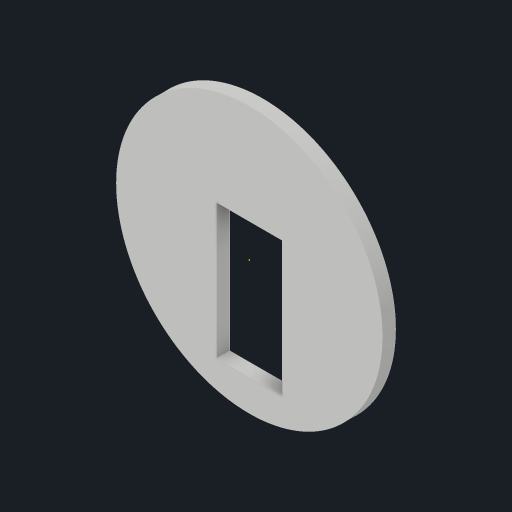
# Autodesk Inventor part: base22
Saved by Autodesk Inventor 2023.4 (Build 274418000, 418)
## iProperties
Created: 2016-02-08
Part Number: base22
Material: Generic
Document SubType Name: Modeling
Designer: Nanjar
Density: 1 g/cm^3
Appearance: Default
Author: Nanjar
Autodesk Inventor part; units mm, degrees
ref_plane "YZ Plane" through (0, 0, 0) normal (1, 0, 0) x (0, 1, 0)
ref_plane "XZ Plane" through (0, 0, 0) normal (0, 1, 0) x (-1, 0, 0)
ref_plane "XY Plane" through (0, 0, 0) normal (0, 0, 1) x (1, 0, 0)
sketch "Sketch1" plane through (0, 0, 0) normal (0, 0, 1) x (1, 0, 0)
  circle A0 centre (0, 0) radius 40
  circle A1 centre (0, 0) radius 5.375
  dimension "d0" = 80
  dimension "d1" = 10.75
  constraints: 2 centre point, 2 coincident
  measures "d0" diameter of A0
  measures "d1" diameter of A1
extrude "Extrusion1" add sketch "Sketch1" along normal blind 4
sketch "Sketch5" plane through (0, 0, 4) normal (0, 0, 1) x (1, 0, 0)
  point P0 (0, 0)
sketch "Sketch7" plane through (0, 0, 4) normal (0, 0, 1) x (1, 0, 0)
  line L0 (-9.9, 10) -> (9.9, 10)
  line L1 (9.9, 10) -> (9.9, -30.6)
  line L2 (9.9, -30.6) -> (-9.9, -30.6)
  line L3 (-9.9, -30.6) -> (-9.9, 10)
  circle A0 centre (0, 0) radius 5.375 projected
  dimension "d19" = 19.8
  dimension "d20" = 40.6
  dimension "d21" = 10
  dimension "d22" = 9.9
  constraints: 8 end point, 2 parallel, 1 horizontal, 1 perpendicular
  measures "d19" distance of L1.end L2.end
  measures "d20" distance of L0.end L1.end
  measures "d21" distance from line of L0 A0.centre
  measures "d22" distance from line of L3 A0.centre
extrude "Extrusion5" cut sketch "Sketch7" against normal blind 4
body "Solid1"
